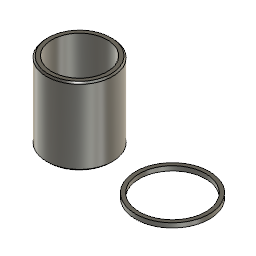
alkane-lamp-connector-pipe-43mm (Autodesk Fusion 360 design; units mm, degrees)
Autodesk Fusion 360 part; units mm, degrees
sketch "Skizze14" plane through (0, 0, 0) normal (0, 0, 1) x (1, 0, 0)
  circle A0 centre (0, 0) radius 18
  circle A1 centre (0, 0) radius 21.45
extrude "Extrusion14" add sketch "Skizze14" along normal blind 50 makes body 1
sketch "Skizze15" plane through (0, 0, 0) normal (0, 0, 1) x (1, 0, 0)
  circle A0 centre (60.5, 0) radius 21.525
  circle A1 centre (60.5, 0) radius 24
extrude "Extrusion15" add sketch "Skizze15" along normal blind 3 separate body makes body 2
chamfer "Fase8" distance 1 angle 45 2 edges at (-19.9984, -7.7567, 50) (-19.9984, -7.7567, 0) on bodies 1
equation "outer_diameter = 43 mm" comment "Nenn-Außendurchmesser des Rohres (43mm)"
equation "outer_clearance = -0.10 mm" comment "Passungsspiel des Außendurchmessers (-0.10mm)"
equation "inner_diameter = 36 mm" comment "Innendurchmesser des Rohres (Kabelkanal)"
equation "pipe_length = 50 mm" comment "Gesamtlänge des Verbindungsrohres"
equation "ring_as_separate_body = 1" comment "Ring als separates Bauteil erzeugen (1 = Ja auf XY-Ebene, 0 = Nein/integriert)"
equation "ring_outer_diameter = 48 mm" comment "Außendurchmesser des Anschlagrings"
equation "ring_inner_diameter = 43 mm" comment "Nenn-Innendurchmesser des separaten Anschlagrings"
equation "ring_inner_clearance = 0.05 mm" comment "Passungsspiel/Aufmaß des Ring-Innendurchmessers (+0.05mm)"
equation "ring_length = 3 mm" comment "Länge des Anschlagrings"
equation "outer_chamfer = 1 mm" comment "Fase an den äußeren Endkanten des Rohres"
equation "d60 = pipe_length"
equation "d62 = ring_length"
equation "d64 = outer_chamfer"
named bodies: "connector-pipe-43mm", "connector-pipe-ring-48mm"
